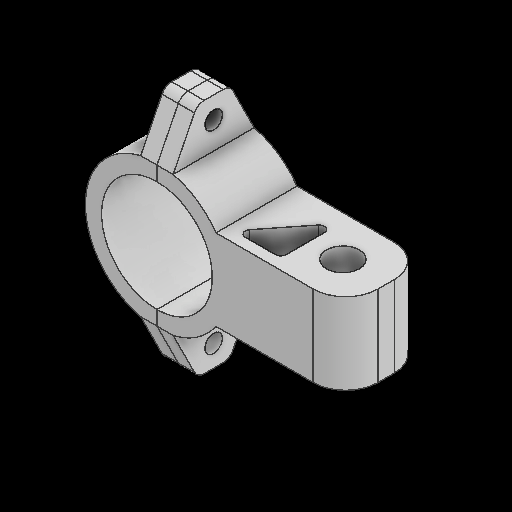
# Autodesk Inventor part: ScreenMount
Saved by Autodesk Inventor 2025.2 (Build 292293000, 293)
## iProperties
Created: 2026-06-24
Part Number: ScreenMount
Material: Generic
Document SubType Name: Modeling
Designer: valer
Density: 1 g/cm^3
Appearance: Default
Author: valer
Autodesk Inventor part; units mm, degrees
ref_plane "YZ Plane" through (0, 0, 0) normal (1, 0, 0) x (0, 1, 0)
ref_plane "XZ Plane" through (0, 0, 0) normal (0, 1, 0) x (-1, 0, 0)
ref_plane "XY Plane" through (0, 0, 0) normal (0, 0, 1) x (1, 0, 0)
sketch "Base" plane through (0, 0, 0) normal (0, 0, 1) x (1, 0, 0)
  circle A0 centre (0, 0) radius 10.25
  circle A1 centre (0, 0) radius 13.25
  line L0 (0, 13.25) -> (0, 21.9059)
  line L1 (0, 21.9059) -> (3, 21.9059)
  line L2 (3, 21.9059) -> (3, 12.9059)
  line L3 (0, -30.6683) -> (0, 30.6683) projected
  line L4 (-18.55, 0) -> (18.55, 0) construction
  line L5 (0, -13.25) -> (0, -21.9059)
  line L6 (0, -21.9059) -> (3, -21.9059)
  line L7 (3, -21.9059) -> (3, -12.9059)
  line L8 (0, 21.9059) -> (-3, 21.9059)
  line L9 (-3, 21.9059) -> (-3, 12.9059)
  line L10 (0, -21.9059) -> (-3, -21.9059)
  line L11 (-3, -21.9059) -> (-3, -12.9059)
  point P0 (0, 10.25)
  point P1 (0, -10.25)
  dimension "d0" = 20.5
  dimension "d1" = 3
  dimension "d2" = 3
  dimension "d3" = 9
  constraints: 20 end point, 8 symmetric about line, 2 centre point, 2 coincident, 2 perpendicular, 2 point on circle, 1 collinear, 1 vertical
  measures "d0" diameter of A0
  measures "d1" radial gap between concentric circles of A0 A1
  measures "d2" distance between parallel lines of L2 L0
  measures "d3" distance of L1.end L2.end
extrude "BaseFeature" add sketch "Base" along normal blind 15 contours A0 L3 A1 | L0 L1 L2 A1 | A1 L7 L6 L3 picked at (12.1399, 0.9799)
extrude "HalfFeature" add sketch "Base" along normal blind 15 separate body contours A0 L3 A1 | A1 L9 L8 L0 | L3 L10 L11 A1 picked at (-12.1594, -0.4118)
sketch "Ears" plane through (3, 12.9059, 0) normal (1, 0, 0) x (0, 0, -1)
  line L0 (0, 0) -> (0, 9) projected
  line L1 (0, 9) -> (-15, 9) projected
  line L2 (-15, 0) -> (-15, 9) projected
  line L3 (0, 0) -> (-15, 0) projected
  line L4 (0, -34.8118) -> (0, -25.8118) projected
  line L5 (0, -25.8118) -> (-15, -25.8118) projected
  line L6 (-15, -34.8118) -> (-15, -25.8118) projected
  line L7 (0, -34.8118) -> (-15, -34.8118) projected
  line L8 (-15, 0) -> (-10.5, 9)
  line L9 (-7.5, -34.8118) -> (-7.5, 9) construction
  line L10 (-15, -23.1559) -> (-15, -2.6559) projected
  line L11 (-15, -12.9059) -> (0, -12.9059) construction
  line L12 (0, -23.1559) -> (0, -2.6559) projected
  line L13 (-15, -25.8118) -> (-10.5, -34.8118)
  line L14 (0, 0) -> (-4.5, 9)
  line L15 (0, -25.8118) -> (-4.5, -34.8118)
  dimension "d9" = 6
  constraints: 12 end point, 6 symmetric about line, 3 midpoint, 1 perpendicular, 1 point on line
  measures "d9" distance of L14.end L8.end
extrude "BaseEarsFeature" cut sketch "Ears" against normal through all contours L14 L1 L0 | L2 L1 L8 | L7 L15 L4 | L13 L7 L6 bodies 1
extrude "HalfEarsFeatrue" cut sketch "Ears" against normal through all contours L14 L1 L0 | L2 L1 L8 | L7 L15 L4 | L13 L7 L6 bodies 2
fillet "EarFilletsFeature" radius 2 8 edges at (1.5, 21.9059, 10.5) (1.5, 21.9059, 4.5) (1.5, -21.9059, 10.5) (1.5, -21.9059, 4.5) (-1.5, 21.9059, 10.5) (-1.5, 21.9059, 4.5) (-1.5, -21.9059, 10.5) (-1.5, -21.9059, 4.5)
sketch "EarMountHoles" plane through (3, 12.9059, 13.7757) normal (1, 0, 0) x (0, 0, -1)
  arc A0 (9.8285, 7.8944) -> (8.0397, 9) centre (8.0397, 7) ccw projected
  line L0 (8.0397, 9) -> (4.5118, 9) projected
  arc A1 (4.5118, 9) -> (2.7229, 7.8944) centre (4.5118, 7) ccw projected
  line L1 (2.7229, 7.8944) -> (-1.2243, 0) projected
  line L2 (13.7757, 0) -> (-1.2243, 0) projected
  line L3 (13.7757, 0) -> (9.8285, 7.8944) projected
  circle A2 centre (6.2757, 5) radius 1.625
  line L4 (8.0397, -34.8118) -> (4.5118, -34.8118) projected
  line L5 (6.2757, -34.8118) -> (6.2757, 9) construction
  line L6 (-1.2243, -23.1559) -> (-1.2243, -2.6559) projected
  line L7 (-1.2243, -12.9059) -> (13.7757, -12.9059) construction
  circle A3 centre (6.2757, -30.8118) radius 1.625
  dimension "d15" = 3.25
  dimension "d16" = 4
  constraints: 4 end point, 3 midpoint, 2 centre point, 1 horizontal, 1 point on line, 1 symmetric about line, 1 other
  measures "d15" diameter of A2
  measures "d16" vertical distance of L0.end A2.centre
extrude "EarMountHolesHalfFeature" cut sketch "EarMountHoles" against normal through all contours A2 | A3 bodies 1
extrude "EarMountHolesOtherHalfFeature" cut sketch "EarMountHoles" against normal blind 10 contours A2 | A3 bodies 2
sketch "MonitorArmMount" plane through (0, 0, 15) normal (0, 0, 1) x (1, 0, 0)
  line L0 (-6.5764, 0) -> (39.4584, 0) projected
  line L1 (0, -30.6683) -> (0, 30.6683) projected
  arc A0 (3, -12.9059) -> (3, 12.9059) centre (0, 0) ccw projected
  line L2 (10.923, -7.5) -> (34.923, -7.5)
  line L3 (34.923, -7.5) -> (34.923, 7.5)
  line L4 (34.923, 7.5) -> (10.923, 7.5)
  point P0 (34.923, 0)
  dimension "d21" = 24
  dimension "d22" = 15
  constraints: 6 end point, 2 point on circle, 1 horizontal, 1 midpoint, 1 parallel, 1 perpendicular, 1 point on line
  measures "d21" distance of L2.start L2.end
  measures "d22" distance of L2.end L3.end
extrude "MonitorArmMountFeature" add sketch "MonitorArmMount" against normal up to surface (15 mm away) bodies 1
fillet "OutsideFilletsFeature" radius 6 2 edges at (34.923, 0, 15) (34.923, 0, 0)
sketch "MonitorMount" plane through (10.923, 7.5, 15) normal (0, 1, 0) x (1, 0, 0)
  arc A0 (24, 9) -> (18, 15) centre (18, 9) ccw projected
  line L0 (0, 15) -> (18, 15) projected
  line L1 (0, 0) -> (0, 15) projected
  line L2 (18, 0) -> (0, 0) projected
  arc A1 (18, 0) -> (24, 6) centre (18, 6) ccw projected
  line L3 (24, 6) -> (24, 9) projected
  circle A2 centre (16, 7.5) radius 3.05
  line L4 (24, 7.5) -> (0, 7.5) construction
  line L5 (0, 0) -> (0, 15) projected
  line L6 (24, 6) -> (24, 9) projected
  point P0 (-10.923, 15)
  dimension "d26" = 6.1
  dimension "d29" = 8
  constraints: 3 midpoint, 2 end point, 1 centre point, 1 perpendicular, 1 point on line
  measures "d26" diameter of A2
  measures "d29" distance of point (24, 7.5) A2.centre
extrude "MonitorMountFeature" cut sketch "MonitorMount" against normal through all contours A2 bodies 1
sketch "MountHoles" plane through (10.923, 7.5, 15) normal (0, 1, 0) x (1, 0, 0)
  circle A0 centre (16, 7.5) radius 3.05 projected
  arc A1 (24, 9) -> (18, 15) centre (18, 9) ccw projected
  line L0 (0, 15) -> (18, 15) projected
  line L1 (0, 0) -> (0, 15) projected
  line L2 (18, 0) -> (0, 0) projected
  arc A2 (18, 0) -> (24, 6) centre (18, 6) ccw projected
  line L3 (24, 6) -> (24, 9) projected
  line L4 (10, 13) -> (1.327, 2)
  line L5 (1.327, 2) -> (10, 2)
  line L6 (-0.673, 0) -> (-0.673, 15) projected
  line L7 (10, 2) -> (10, 13)
  line L8 (6.1797, 13) -> (1.327, 6.8453)
  line L9 (1.327, 6.8453) -> (1.327, 13)
  line L10 (1.327, 13) -> (6.1797, 13)
  line L11 (18, 0) -> (0, 0) projected
  line L12 (0, 15) -> (18, 15) projected
  line L13 (24, 6) -> (24, 9) projected
  line L14 (10, 13) -> (6.1797, 13)
  line L15 (1.327, 2) -> (1.327, 6.8453)
  point P0 (-10.923, 15)
  dimension "d30" = 3
  dimension "d31" = 2
  dimension "d32" = 2
  dimension "d33" = 2
  dimension "d34" = 6
  constraints: 16 end point, 5 parallel, 3 perpendicular, 2 collinear
  measures "d30" distance between parallel lines of L8 L4
  measures "d31" distance between parallel lines of L2 L5
  measures "d32" distance between parallel lines of L0 L10
  measures "d33" distance between parallel lines of L6 L15
  measures "d34" distance from line of A0.centre L7
extrude "MountHolesFeature" cut sketch "MountHoles" against normal through all contours L7 L5 L4 bodies 1
fillet "InsideFilletsFeature" radius 1 3 edges at (20.923, 0, 13) (12.25, 0, 13) (20.923, 0, 2)
equation "\"d32\" = d31"
equation "\"d33\" = d31"
